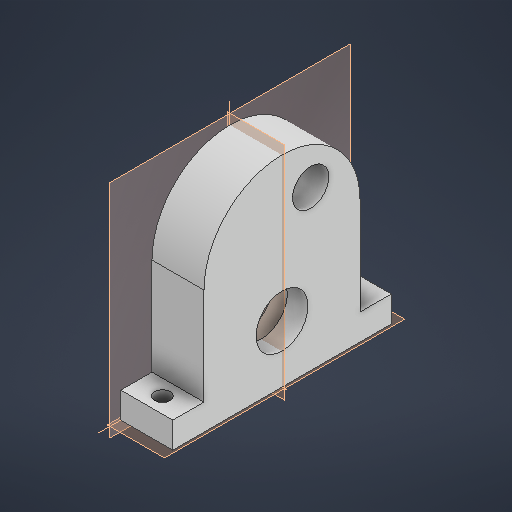
# Autodesk Inventor part: support_arriere_droite
Saved by Autodesk Inventor 2027.1 (Build 311270010, 270A)
## iProperties
Created: 2026-09-09
Part Number: support_arriere_droite
Material: Generic
Document SubType Name: Modeling
Designer: thiag
Density: 1 g/cm^3
Appearance: Default
Author: thiag
Autodesk Inventor part; units mm, degrees
sketch "Sketch1" plane through (0, 0, 0) normal (1, 0, 0) x (0, 1, 0)
  circle A0 centre (30.5, -5.5) radius 3.5
  line L0 (11, 15) -> (5, 15)
  line L1 (5, -15) -> (11, -15)
  line L2 (0, -21) -> (5, -21)
  line L3 (5, -21) -> (5, -15)
  line L4 (0, 21) -> (5, 21)
  line L5 (5, 21) -> (5, 15)
  line L6 (-7.7302, 0) -> (46.3815, 0) projected
  line L7 (0, 29.4) -> (0, -29.4) projected
  line L8 (0, 21) -> (0, -21)
  line L9 (11, -15) -> (23.6512, -15)
  line L10 (11, 15) -> (23.6512, 15)
  arc A1 (23.6512, -15) -> (23.6512, 15) centre (23.6512, 0) ccw
  circle A2 centre (11, 0) radius 5
  point P0 (2.5, -21)
  dimension "d7" = 7
  dimension "d45" = 21
  dimension "d64" = 5
  dimension "d65" = 21
  dimension "d66" = 5
  dimension "d67" = 15
  dimension "d69" = 5.5
  dimension "d73" = 0
  dimension "d74" = 30.5
  dimension "d75" = 10
  dimension "d76" = 0
  dimension "d77" = 11
  dimension "d78" = 15
  dimension "d79" = 15
  dimension "d80" = 23.6512
  constraints: 18 end point, 3 centre point, 3 horizontal, 2 point on circle, 1 midpoint, 1 parallel, 1 point on line
  measures "d7" diameter of A0
  measures "d45" distance between parallel lines of L6 L2
  measures "d64" distance between parallel lines of L7 L3
  measures "d65" distance between parallel lines of L4 L6
  measures "d66" distance between parallel lines of L7 L5
  measures "d67" distance from line of L6 L1.start
  measures "d69" distance from line of A0.centre L6
  measures "d73" distance between parallel lines of L7 L8
  measures "d74" distance from line of L8 A0.centre
  measures "d75" diameter of A2
  measures "d76" distance from line of L6 A2.centre
  measures "d77" distance from line of L8 A2.centre
  measures "d78" distance between parallel lines of L6 L10
  measures "d79" radius of A1
  measures "d80" distance from line of L8 A1.centre
extrude "Extrusion1" add sketch "Sketch1" along normal blind 10 contours L10 A1 L6 A2 L7 L4 L5 L0 | A1 L9 L1 L3 L2 L7 L6 A2
sketch "Sketch4" plane through (10, 0, 0) normal (1, 0, 0) x (0, 0, -1)
  circle A0 centre (0, 11) radius 9.5
  line L0 (-29.4, 0) -> (29.4, 0) projected
  line L1 (0, -7.7302) -> (0, 46.3815) projected
  point P0 (0, 0)
  dimension "d56" = 19
  dimension "d58" = 11
  dimension "d59" = 0
  constraints: 1 centre point
  measures "d56" diameter of A0
  measures "d58" distance from line of L0 A0.centre
  measures "d59" distance from line of L1 A0.centre
extrude "Extrusion2" cut sketch "Sketch4" along normal blind 6 from surface at -10
sketch "Sketch6" plane through (0, 5, -15) normal (0, 1, 0) x (1, 0, 0)
  circle A0 centre (5, 3) radius 1.5
  line L0 (12, -15) -> (-2, -15) projected
  circle A1 centre (5, -33) radius 1.5
  line L1 (0, -30) -> (0, -36) projected
  line L2 (0, 6) -> (0, 0) projected
  point P0 (0, -15)
  point P1 (0, -33)
  point P2 (0, 3)
  dimension "d81" = 3
  dimension "d82" = 18
  dimension "d83" = 3
  dimension "d84" = 18
  dimension "d85" = 5
  dimension "d86" = 5
  constraints: 2 centre point, 2 midpoint
  measures "d81" diameter of A0
  measures "d82" distance from line of L0 A0.centre
  measures "d83" diameter of A1
  measures "d84" distance from line of L0 A1.centre
  measures "d85" distance of point (0, -33) A1.centre
  measures "d86" distance of point (0, 3) A0.centre
extrude "Extrusion3" cut sketch "Sketch6" against normal blind 5
sketch "Sketch7" plane through (0, 0, 0) normal (-1, 0, 0) x (0, 0, 1)
  circle A0 centre (-5.5, 30.5) radius 5
  line L0 (21, 0) -> (-21, 0) projected
  line L1 (0, -7.7302) -> (0, 46.3815) projected
  point P0 (0, 0)
  dimension "d89" = 10
  dimension "d90" = 30.5
  dimension "d91" = 5.5
  constraints: 1 centre point
  measures "d89" diameter of A0
  measures "d90" distance from line of L0 A0.centre
  measures "d91" distance from line of L1 A0.centre
extrude "Extrusion4" cut sketch "Sketch7" against normal blind 4
body "Solid1"
